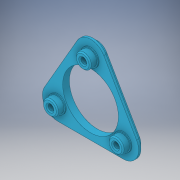
# Autodesk Inventor part: Bottom
Saved by Autodesk Inventor 2019.1 (Build 231200000, 200)
## iProperties
Created: 2019-01-01
Part Number: Bottom
Material: Generisch
Document SubType Name: Modeling
Designer: JochenAlt
Density: 1 g/cm^3
Appearance: Vorgabe
Author: JochenAlt
Autodesk Inventor part; units mm, degrees
ref_plane "YZ Plane" through (0, 0, 0) normal (1, 0, 0) x (0, 1, 0)
ref_plane "XZ Plane" through (0, 0, 0) normal (0, 1, 0) x (-1, 0, 0)
ref_plane "XY Plane" through (0, 0, 0) normal (0, 0, 1) x (1, 0, 0)
sketch "Skizze1" plane through (0, 0, 0) normal (0, 0, 1) x (1, 0, 0)
  circle A0 centre (0, 0) radius 17 construction
  line L0 (0, 32.0325) -> (0, -25.245) construction
  circle A1 centre (0, 17) radius 1.3
  circle A2 centre (14.7224, -8.5) radius 1.3
  circle A3 centre (-14.7224, -8.5) radius 1.3
  line L1 (0, 17) -> (14.7224, -8.5) construction
  line L2 (-14.7224, -8.5) -> (14.7224, -8.5) construction
  line L3 (-14.7224, -8.5) -> (0, 17) construction
  line L4 (5.9323, 20.425) -> (20.6547, -5.075)
  line L5 (14.7224, -15.35) -> (-14.7224, -15.35)
  line L6 (-20.6547, -5.075) -> (-5.9323, 20.425)
  arc A4 (-20.6547, -5.075) -> (-14.7224, -15.35) centre (-14.7224, -8.5) ccw
  arc A5 (14.7224, -15.35) -> (20.6547, -5.075) centre (14.7224, -8.5) ccw
  arc A6 (5.9323, 20.425) -> (-5.9323, 20.425) centre (0, 17) ccw
  circle A7 centre (0, 17) radius 3.35
  circle A8 centre (-14.7224, -8.5) radius 3.35
  circle A9 centre (14.7224, -8.5) radius 3.35
  circle A10 centre (0, 17) radius 3.85
  circle A11 centre (14.7224, -8.5) radius 3.85
  circle A12 centre (-14.7224, -8.5) radius 3.85
  circle A13 centre (0, 0) radius 12.5
  circle A14 centre (0, 17) radius 2.5
  circle A15 centre (-14.7224, -8.5) radius 2.5
  circle A16 centre (14.7224, -8.5) radius 2.5
  point P0 (0, 13.15)
  point P1 (0, 12.5)
  dimension "d19" = 12.5
  dimension "d1" = 2.6
  dimension "d2" = 17
  dimension "d3" = 0.5
  dimension "d4" = 6.7
  dimension "d5" = 3
  dimension "d16" = 5
  constraints: 15 centre point, 14 coincident, 12 end point, 9 equal radius, 9 point on circle, 6 tangent, 3 point on line, 2 equal length, 2 vertical alignment, 5 other
  measures "d1" diameter of A1
  measures "d2" radius of A0
  measures "d4" diameter of A7
  measures "d16" diameter of A14
extrude "Extrusion1" add sketch "Skizze1" along normal blind 3 contours L4 A5 L5 A4 L6 A6 | A7 | A8 | A9 | A10 | A11 | A12 | A14 | A15 | A16
extrude "Extrusion2" add sketch "Skizze1" along normal blind 0.5 from surface at 3 contours A7 | A8 | A9 | A10 | A11 | A12 | A14 | A15 | A16
extrude "Extrusion3" add sketch "Skizze1" along normal blind 3 from surface at 3.5 contours A7 | A8 | A9 | A14 | A15 | A16
chamfer "Fase1" distance 0.5 angle 45 6 edges at (-3.35, 17, 6.5) (-18.0724, -8.5, 6.5) (11.3724, -8.5, 6.5) (-1.3, 17, 6.5) (-16.0224, -8.5, 6.5) (13.4224, -8.5, 6.5)
extrude "Extrusion4" cut sketch "Skizze1" along normal blind 2 contours A14 | A15 | A16
chamfer "Fase2" distance 2 angle 45 6 edges at (0, -15.35, 0) (-20.6547, -11.925, 0) (-13.2935, 7.675, 0) (0, 23.85, 0) (13.2935, 7.675, 0) (20.6547, -11.925, 0)
